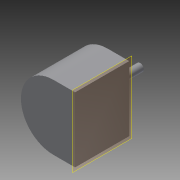
# Autodesk Inventor part: motor
Saved by Autodesk Inventor 2014 (Build 180170000, 170)
## iProperties
Created: 2014-11-30
Part Number: motor
Material: Generic
Document SubType Name: Modeling
Designer: ph1140784
Density: 1 g/cm^3
Appearance: Default
Author: ph1140784
Autodesk Inventor part; units mm, degrees
ref_plane "XZ Plane" through (0, 0, 0) normal (0, 1, 0) x (-1, 0, 0)
ref_plane "XY Plane" through (0, 0, 0) normal (0, 0, 1) x (1, 0, 0)
sketch "Sketch1" plane through (0, 0, 0) normal (0, 1, 0) x (-1, 0, 0)
  circle A0 centre (0, 0) radius 30
  dimension "d0" = 60
  constraints: 1 centre point, 1 coincident
  measures "d0" diameter of A0
extrude "Extrusion1" add sketch "Sketch1" along normal blind 50
sketch "Sketch2" plane through (0, 50, 0) normal (0, 1, 0) x (1, 0, 0)
  circle A0 centre (0, 0) radius 30 projected
  circle A1 centre (0, 0) radius 3.5
  dimension "d3" = 7
  constraints: 1 centre point, 1 coincident
  measures "d3" diameter of A1
extrude "Extrusion2" add sketch "Sketch2" along normal blind 30 contours A1
ref_plane "Work Plane1" through (30, 0, 0) normal (1, 0, 0) x (0, 1, 0)
sketch "Sketch3" plane through (30, 0, 0) normal (1, 0, 0) x (0, 1, 0)
  line L0 (50, -30) -> (50, 30) projected
  line L1 (0, 30) -> (0, -30) projected
  line L2 (0, -30) -> (50, -30)
  line L3 (50, -30) -> (50, 30)
  line L4 (50, 30) -> (0, 30)
  line L5 (0, 30) -> (0, -30)
  point P0 (0, 0)
  constraints: 8 end point, 2 parallel, 1 horizontal, 1 perpendicular
extrude "Extrusion3" add sketch "Sketch3" against normal up to next
sketch "Sketch4" plane through (30, 0, 0) normal (1, 0, 0) x (0, 0, -1)
  line L0 (30, 0) -> (-30, 0) projected
  line L1 (30, 50) -> (30, 0) projected
  line L2 (-30, 50) -> (30, 50) projected
  line L3 (-30, 0) -> (-30, 50) projected
  point P0 (0, 0)
ref_plane "Work Plane2" through (20, 0, 0) normal (1, 0, 0) x (0, 0, -1)
extrude "Extrusion4" cut sketch "Sketch4" against normal blind 10
body "Solid1"
